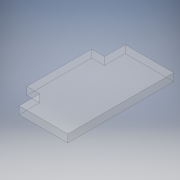
# Autodesk Inventor part: bottom perspex
Saved by Autodesk Inventor 2019 (Build 230136000, 136)
## iProperties
Created: 2020-02-17
Part Number: bottom perspex
Material: Generic
Document SubType Name: Modeling
Designer: craggles
Density: 1 g/cm^3
Appearance: Polycarbonate - Clear
Author: craggles
Autodesk Inventor part; units mm, degrees
ref_plane "YZ Plane" through (0, 0, 0) normal (1, 0, 0) x (0, 1, 0)
ref_plane "XZ Plane" through (0, 0, 0) normal (0, 1, 0) x (-1, 0, 0)
ref_plane "XY Plane" through (0, 0, 0) normal (0, 0, 1) x (1, 0, 0)
sketch "Sketch1" plane through (0, 0, 0) normal (0, 1, 0) x (-1, 0, 0)
  line L0 (-42.845, -43.5625) -> (-42.845, 65.5625)
  line L1 (33.4911, -43.5625) -> (33.4911, 65.5625)
  line L2 (33.4911, 30) -> (33.4911, -8)
  line L3 (-42.845, -8) -> (-42.845, 30)
  line L4 (-42.845, -43.5625) -> (-42.845, 65.5625)
  line L5 (-42.845, 30) -> (-17.845, 30)
  line L6 (-17.845, 30) -> (-17.845, -8)
  line L7 (-17.845, -8) -> (-42.845, -8)
  line L8 (-42.845, -8) -> (-42.845, 30)
  line L9 (33.4911, 30) -> (8.4911, 30)
  line L10 (8.4911, 30) -> (8.4911, -8)
  line L11 (8.4911, -8) -> (33.4911, -8)
  line L12 (33.4911, -8) -> (33.4911, 30)
  line L13 (-17.845, 30) -> (-17.845, -8)
  line L14 (8.4911, -8) -> (8.4911, 30)
  line L15 (-17.845, 30) -> (-15.845, 30)
  line L16 (-15.845, 30) -> (-15.845, -8)
  line L17 (-15.845, -8) -> (-17.845, -8)
  line L18 (-17.845, -8) -> (-17.845, 30)
  line L19 (8.4911, 30) -> (6.4911, 30)
  line L20 (6.4911, 30) -> (6.4911, -8)
  line L21 (6.4911, -8) -> (8.4911, -8)
  line L22 (8.4911, -8) -> (8.4911, 30)
  line L23 (-15.845, -8) -> (-15.845, 30)
  line L24 (6.4911, 30) -> (6.4911, -8)
  line L25 (-15.845, -8) -> (-15.845, 30)
  line L26 (-15.845, 30) -> (-15.845, -8)
  line L27 (0, 22) -> (0, 40.5625)
  line L28 (-17.845, -8) -> (0, -8)
  line L29 (0, -8) -> (0, 30)
  line L30 (0, 30) -> (-17.845, 30)
  line L31 (-17.845, 30) -> (-17.845, -8)
  line L32 (5, 22) -> (5, 0)
  line L33 (0, 22) -> (5, 22)
  line L34 (5, 22) -> (5, 0)
  line L35 (5, 0) -> (0, 0)
  line L36 (0, 0) -> (0, 22)
  line L37 (1.5, 31.5) -> (-17.345, 31.5)
  line L38 (-17.345, 31.5) -> (-17.345, -9.5)
  line L39 (-17.345, -9.5) -> (1.5, -9.5)
  line L40 (1.5, -9.5) -> (1.5, 31.5)
  line L41 (6.5, 23.5) -> (0, 23.5)
  line L42 (0, 23.5) -> (0, -1.5)
  line L43 (0, -1.5) -> (6.5, -1.5)
  line L44 (6.5, -1.5) -> (6.5, 23.5)
  point P0 (-45.9471, 11)
  point P1 (-45.845, 65.5625)
  point P2 (36.4911, 65.5625)
  point P3 (-42.845, 11)
  point P4 (-42.845, 11)
  dimension "d0" = 38
  dimension "d1" = 25
  dimension "d2" = 38
  dimension "d3" = 25
  dimension "d4" = 2
  dimension "d5" = 2
  dimension "d6" = 1.5
  dimension "d7" = 1.5
  dimension "d8" = 1.5
  dimension "d9" = 1.5
  dimension "d10" = 1.5
  dimension "d11" = 1.5
  dimension "d12" = 1.5
  constraints: 84 end point, 19 parallel, 8 horizontal, 8 perpendicular, 3 point on line, 1 coincident, 1 midpoint, 12 other
  measures "d0" distance of L9.start L2.end
  measures "d1" distance of L6.end L7.end
  measures "d2" distance of L6.start L6.end
  measures "d3" distance of L11.end L11.start
  measures "d4" distance of L17.start L28.start
  measures "d5" distance of L21.end L21.start
  measures "d6" distance between parallel lines of L38 L16
  measures "d7" distance between parallel lines of L39 L28
  measures "d8" distance between parallel lines of L40 L29
  measures "d9" distance between parallel lines of L37 L30
  measures "d10" distance between parallel lines of L33 L41
  measures "d11" distance between parallel lines of L32 L44
  measures "d12" distance between parallel lines of L43 L35
extrude "Extrusion1" add sketch "Sketch1" along normal blind 3 contours L38 L15 L16 L17 | L17 L28 L29 L43 L40 L39 L38 | L38 L37 L27 L30 L15 | L16 L30 L27 L29 L28 | L27 L37 L40 L41 | L29 L35 L40 L43 | L40 L35 L32 L33 L41 L20 L43 | L41 L40 L33 L27 | L29 L33 L40 L35 | L40 L33 L32 L35 | L20 L41 L44 L43
equation "\"d8\" = d7"
equation "\"d9\" = d7"
equation "\"d10\" = d9"
equation "\"d11\" = d7"
equation "\"d12\" = d7"
body "Solid1"
